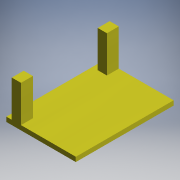
# Autodesk Inventor part: Upper_leg-01
Saved by Autodesk Inventor 2017 (Build 210142000, 142)
## iProperties
Part Number: Upper_leg-01
Material: Generic
Document SubType Name: Modeling
Designer: alex-
Appearance: Canary
Author: alex-
Autodesk Inventor part; units mm, degrees
ref_plane "YZ Plane" through (0, 0, 0) normal (1, 0, 0) x (0, 1, 0)
ref_plane "XZ Plane" through (0, 0, 0) normal (0, 1, 0) x (-1, 0, 0)
ref_plane "XY Plane" through (0, 0, 0) normal (0, 0, 1) x (1, 0, 0)
sketch "Sketch8" plane through (0, 0, 0) normal (0, 1, 0) x (-1, 0, 0)
  line L0 (19, 26.75) -> (-19, 26.75)
  line L1 (-19, 26.75) -> (-19, -26.75)
  line L2 (-19, -26.75) -> (19, -26.75)
  line L3 (19, -26.75) -> (19, 26.75)
  point P0 (0, 0)
  point P1 (0, 26.75)
  point P2 (19, 0)
  dimension "d31" = 38
  dimension "d32" = 53.5
  constraints: 8 end point, 2 midpoint, 2 parallel, 1 horizontal, 1 horizontal alignment, 1 perpendicular, 1 vertical alignment
  measures "d31" distance of L0.start L0.end
  measures "d32" distance of L2.end L0.start
extrude "Extrusion8" add sketch "Sketch8" along normal blind 2.5
sketch "Sketch9" plane through (0, 2.5, 0) normal (0, 1, 0) x (1, 0, 0)
  line L0 (-16, -26.75) -> (-11, -26.75)
  line L1 (-11, -26.75) -> (-11, -20.25)
  line L2 (-11, -20.25) -> (-16, -20.25)
  line L3 (-16, -20.25) -> (-16, -26.75)
  line L4 (-16, 20.25) -> (-11, 20.25)
  line L5 (-11, 20.25) -> (-11, 26.75)
  line L6 (-11, 26.75) -> (-16, 26.75)
  line L7 (-16, 26.75) -> (-16, 20.25)
  line L8 (-19, -26.75) -> (19, -26.75) projected
  line L9 (19, 26.75) -> (-19, 26.75) projected
  line L10 (-19, 26.75) -> (-19, -26.75) projected
  point P0 (0, 0)
  point P1 (-13.5, -26.75)
  point P2 (-13.5, 26.75)
  dimension "d35" = 6.5
  dimension "d36" = 5
  dimension "d38" = 8
  constraints: 16 end point, 4 parallel, 2 equal length, 2 horizontal, 2 midpoint, 2 perpendicular, 2 point on line, 1 vertical alignment
  measures "d35" distance of L2.end L0.start
  measures "d36" distance of L1.end L2.end
  measures "d38" distance between parallel lines of L1 L10
extrude "Extrusion9" add sketch "Sketch9" along normal blind 20
equation "\"d31\" = s_height"
equation "\"d32\" = s_width + 2 * s_land"
equation "\"d33\" = 0.5 * b_mat_thickness"
equation "\"d35\" = s_land"
equation "\"d36\" = b_mat_thickness"
equation "\"d38\" = s_land_dist_top"
equation "\"d39\" = s_depth"
equation "\"s_height\" = 38"
equation "\"s_width\" = 40.5"
equation "\"s_land\" = 6.5"
equation "\"b_mat_thickness\" = 5"
equation "\"s_land_dist_top\" = 8"
equation "\"s_depth\" = 20"
body "Solid2"
